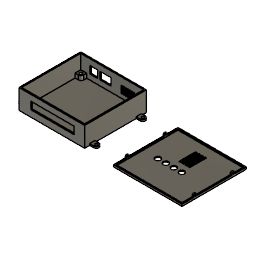
Carte ESP32 4 Relais (Autodesk Fusion 360 design; units mm, degrees)
Autodesk Fusion 360 part; units mm, degrees
note: some values were not read from the file. Chosen so that the rebuilt part matches the saved one: which bodies a step acts on; a direction. Set by a fixed rule: which sketch regions a step uses.
sketch "Esquisse1" plane through (0, 0, 0) normal (0, 0, 1) x (1, 0, 0)
  line L0 (47.5, -44.5) -> (-47.5, -44.5)
  line L1 (-47.5, -44.5) -> (-47.5, 44.5)
  line L2 (-47.5, 44.5) -> (47.5, 44.5)
  line L3 (47.5, 44.5) -> (47.5, -44.5)
  line L4 (47.5, -44.5) -> (-47.5, 44.5) construction
  line L5 (-47.5, -44.5) -> (47.5, 44.5) construction
  line L6 (49.5, -46.5) -> (-49.5, -46.5)
  line L7 (-49.5, -46.5) -> (-49.5, 46.5)
  line L8 (-49.5, 46.5) -> (49.5, 46.5)
  line L9 (49.5, 46.5) -> (49.5, -46.5)
  circle A0 centre (55.5, -35) radius 4
  line L10 (55.5, -39) -> (49.5, -39)
  line L11 (55.5, -31) -> (49.5, -31)
  circle A1 centre (55.5, 35) radius 4
  line L12 (55.5, -35) -> (55.5, 39) construction
  line L13 (60, 0) -> (0, 0) construction
  line L14 (55.5, 39) -> (49.5, 39)
  line L15 (55.5, 31) -> (49.5, 31)
  circle A2 centre (-55.5, -35) radius 4
  circle A3 centre (-55.5, 35) radius 4
  line L16 (-55.5, -35) -> (-55.5, 35) construction
  line L17 (-55.5, -39) -> (-49.5, -39)
  line L18 (-55.5, -31) -> (-49.5, -31)
  line L19 (-55.5, 31) -> (-49.5, 31)
  line L20 (-55.5, 39) -> (-49.5, 39)
  circle A4 centre (-55.5, 35) radius 2
  circle A5 centre (55.5, -35) radius 2
  circle A6 centre (-55.5, -35) radius 2
  circle A7 centre (55.5, 35) radius 2
  dimension "d1" = 95
  dimension "d2" = 89
  dimension "d3" = -2
  dimension "d56" = 8
  dimension "d59" = 8
  dimension "d60" = 70
  dimension "d61" = 8
  dimension "d62" = 8
  dimension "d63" = 6
  dimension "d64" = 6
  dimension "d65" = 4
  dimension "d66" = 4
  dimension "d67" = 4
  dimension "d68" = 4
  constraint horizontal L0
  constraint perpendicular L0 L1
  constraint parallel L0 L2
  constraint parallel L1 L3
  constraint coincident L4 L13.end
  constraint coincident L5 L13.end
  constraint coincident L13.end origin
  constraint coincident A0 L10.start
  constraint coincident L9 L10.end
  constraint perpendicular L9 L10
  constraint coincident A0 L11.start
  constraint coincident L9 L11.end
  constraint perpendicular L9 L11
  constraint coincident A0.centre L12.start
  constraint perpendicular L11 L12
  constraint coincident A1 L12.end
  constraint horizontal L13
  constraint symmetric A0 A1 L13
  constraint coincident L9 L14.end
  constraint tangent A1 L14
  constraint coincident A1 L15.start
  constraint coincident L12 L15.start
  constraint coincident L9 L15.end
  constraint perpendicular L9 L15
  constraint coincident A2.centre L16.start
  constraint coincident A3.centre L16.end
  constraint vertical L16
  constraint coincident A2 L17.start
  constraint coincident L7 L17.end
  constraint perpendicular L7 L17
  constraint coincident A2 L18.start
  constraint coincident L16 L18.start
  constraint coincident L7 L18.end
  constraint perpendicular L7 L18
  constraint coincident A3 L19.start
  constraint coincident L16 L19.start
  constraint coincident L7 L19.end
  constraint perpendicular L7 L19
  constraint coincident A3 L20.start
  constraint coincident L7 L20.end
  constraint perpendicular L7 L20
  constraint concentric A2 A6
  constraint concentric A1 A7
  measures "d1" distance of L1.end L2.end
  measures "d2" distance of L0.end L1.end
  measures "d56" diameter of A0
  measures "d59" diameter of A1
  measures "d60" distance of A0.centre A1.centre
  measures "d61" diameter of A2
  measures "d62" diameter of A3
  measures "d63" distance of L9 A0.centre
  measures "d64" distance of L7 L16
  measures "d65" diameter of A4
  measures "d66" diameter of A5
  measures "d67" diameter of A6
  measures "d68" diameter of A7
extrude "Extrusion1" add sketch "Esquisse1" along normal blind 2 contours L0 L1 L2 L3 makes body 1
extrude "Extrusion8" add sketch "Esquisse1" along normal blind 2.5 separate body contours L9 A0 L10 L11 | L7 A2 L17 L18 | A0 | A2 | L9 A1 L14 L15 | L7 A3 L19 L20 | A1 | A3 makes body 2 at (50.8333, -35, 0) makes body 3 at (50.8333, 35, 2.5) makes body 4 at (-50.8333, 35, 0) makes body 5 at (-50.8333, -35, 0)
extrude "Extrusion2" add sketch "Esquisse1" along normal blind 30 contours L6 L7 L8 L9 bodies 1 2 3 4 5
sketch "Esquisse2" plane through (0, -46.5, 0) normal (0, -1, 0) x (1, 0, 0)
  line L0 (-49.5, 0) -> (49.5, 0)
  line L1 (49.5, 0) -> (49.5, 30)
  line L2 (49.5, 30) -> (-49.5, 30)
  line L3 (-49.5, 30) -> (-49.5, 0)
  line L4 (-31.5, 0) -> (33.5, 0)
  line L5 (33.5, 0) -> (33.5, 21)
  line L6 (33.5, 21) -> (-31.5, 21)
  line L7 (-31.5, 21) -> (-31.5, 0)
  line L8 (-31.5, 10) -> (33.5, 10)
  dimension "d8" = 18
  dimension "d9" = 65
  dimension "d11" = 10
  dimension "d135" = 11
  constraint horizontal L4
  constraint vertical L5
  constraint horizontal L6
  constraint vertical L7
  constraint coincident L0 L4.start
  constraint coincident L7 L8.start
  constraint coincident L5 L8.end
  constraint perpendicular L5 L8
  measures "d8" distance of L3 L7
  measures "d9" distance of L5.end L6.end
  measures "d11" distance of L4 L8
  measures "d135" distance of L6 L8
extrude "Extrusion3" cut sketch "Esquisse2" against normal up to surface (2 mm away) contours L5 L6 L7 L8 bodies 1
sketch "Esquisse3" plane through (0, 46.5, 0) normal (0, 1, 0) x (-1, 0, 0)
  line L0 (-49.5, 0) -> (49.5, 0)
  line L1 (49.5, 0) -> (49.5, 30)
  line L2 (49.5, 30) -> (-49.5, 30)
  line L3 (-49.5, 30) -> (-49.5, 0)
  line L4 (33.5, 0) -> (2, 0)
  line L5 (2, 0) -> (2, 21)
  line L6 (2, 21) -> (33.5, 21)
  line L7 (33.5, 21) -> (33.5, 0)
  line L8 (18.5, 21) -> (22, 21)
  line L9 (22, 21) -> (22, 0)
  line L10 (22, 0) -> (18.5, 0)
  line L11 (18.5, 0) -> (18.5, 21)
  line L12 (2, 10) -> (33.5, 10)
  dimension "d14" = 16
  dimension "d18" = 3.5
  dimension "d19" = 10
  dimension "d137" = 11.5
  dimension "d138" = 16.5
  dimension "d144" = 11
  constraint horizontal L4
  constraint vertical L5
  constraint horizontal L6
  constraint vertical L7
  constraint coincident L0 L4.start
  constraint horizontal L8
  constraint vertical L9
  constraint horizontal L10
  constraint vertical L11
  constraint coincident L6 L8.start
  constraint coincident L5 L12.start
  constraint coincident L7 L12.end
  constraint perpendicular L7 L12
  measures "d14" distance of L1 L7
  measures "d18" distance of L9 L11
  measures "d19" distance of L4 L12
  measures "d137" distance of L7 L9
  measures "d138" distance of L5 L11
  measures "d144" distance of L6 L12
extrude "Extrusion4" cut sketch "Esquisse3" against normal up to surface (2 mm away) contours L5 L6 L11 L12 | L6 L7 L9 L12 bodies 1
sketch "Esquisse4" plane through (0, 0, 2) normal (0, 0, 1) x (-1, 0, 0)
  line L0 (-47.5, -44.5) -> (47.5, -44.5)
  line L1 (47.5, -44.5) -> (47.5, 44.5)
  line L2 (47.5, 44.5) -> (-47.5, 44.5)
  line L3 (31.5, 44.5) -> (31.5, 46.5)
  line L4 (31.5, 46.5) -> (-33.5, 46.5)
  line L5 (-33.5, 46.5) -> (-33.5, 44.5)
  line L6 (-47.5, 44.5) -> (-47.5, -44.5)
  circle A0 centre (-42.5, 40) radius 4
  circle A1 centre (42.5, 40) radius 4
  line L7 (0, -48) -> (0, 48) construction
  circle A2 centre (-42.5, -40) radius 4
  circle A3 centre (42.5, -40) radius 4
  line L8 (-58.0065, 0) -> (65, 0) construction
  line L9 (18.5, -44.5) -> (2, -44.5)
  line L10 (2, -44.5) -> (2, -46.5)
  line L11 (2, -46.5) -> (18.5, -46.5)
  line L12 (18.5, -46.5) -> (18.5, -44.5)
  line L13 (33.5, -44.5) -> (22, -44.5)
  line L14 (22, -44.5) -> (22, -46.5)
  line L15 (22, -46.5) -> (33.5, -46.5)
  line L16 (33.5, -46.5) -> (33.5, -44.5)
  line L17 (-33.5, 44.5) -> (31.5, 44.5)
  line L18 (42.5, -36) -> (47.5, -36)
  line L19 (38.5, -40.0091) -> (38.5102, -44.5)
  line L20 (-42.5, -36) -> (-47.5, -36)
  line L21 (-38.5, -40) -> (-38.5, -44.5)
  line L22 (-42.4542, 36.0003) -> (-47.5, 35.9425)
  line L23 (-38.5, 40.0021) -> (-38.5024, 44.5)
  line L24 (42.5, 36) -> (47.5, 36)
  line L25 (38.5, 39.9891) -> (38.4877, 44.5)
  circle A4 centre (-42.5, 40) radius 2.3
  circle A5 centre (42.5, 40) radius 2.3
  circle A6 centre (42.5, -40) radius 2.3
  circle A7 centre (-42.5, -40) radius 2.3
  dimension "d22" = 85
  dimension "d23" = 85
  dimension "d24" = 8
  dimension "d25" = 8
  dimension "d26" = 8
  dimension "d27" = 8
  dimension "d37" = 80
  dimension "d140" = 4.6
  dimension "d141" = 4.6
  dimension "d142" = 4.6
  dimension "d143" = 4.6
  constraint midpoint L7 origin
  constraint perpendicular L4 L7
  constraint symmetric A0.centre A1.centre L7
  constraint symmetric L7 A2.centre A3.centre
  constraint perpendicular L6 L8
  constraint symmetric A0.centre A2.centre L8
  constraint coincident origin L8
  constraint coincident A3 L18.start
  constraint coincident L1 L18.end
  constraint perpendicular L1 L18
  constraint coincident A3 L19.start
  constraint coincident L0 L19.end
  constraint tangent A3 L19
  constraint coincident A2 L20.start
  constraint coincident L6 L20.end
  constraint perpendicular L6 L20
  constraint coincident A2 L21.start
  constraint coincident L0 L21.end
  constraint perpendicular L0 L21
  constraint coincident A0 L22.start
  constraint coincident L6 L22.end
  constraint tangent A0 L22
  constraint coincident A0 L23.start
  constraint coincident L2 L23.end
  constraint tangent A0 L23
  constraint coincident L1 L24.end
  constraint perpendicular L1 L24
  constraint coincident A1 L25.start
  constraint coincident L2 L25.end
  constraint tangent A1 L25
  constraint coincident A1 L24.start
  constraint concentric A0 A4
  constraint concentric A1 A5
  constraint concentric A3 A6
  constraint concentric A2 A7
  measures "d22" distance of A0.centre A1.centre
  measures "d23" distance of A2.centre A3.centre
  measures "d24" diameter of A0
  measures "d25" diameter of A1
  measures "d26" diameter of A2
  measures "d27" diameter of A3
  measures "d37" distance of A0.centre A2.centre
  measures "d140" diameter of A4
  measures "d141" diameter of A7
  measures "d142" diameter of A5
  measures "d143" diameter of A6
extrude "Extrusion5" add sketch "Esquisse4" along normal blind 6.5 contours L0 L6 A2 L20 L21 | A2 | L2 L6 A0 L22 L23 | A0 | L0 L1 A3 L18 L19 | A3 | L1 L2 A1 L24 L25 | A1 bodies 1
sketch "Esquisse6" plane through (0, 46.5, 0) normal (0, 1, 0) x (-1, 0, 0)
  line L0 (2, 21) -> (18.5, 21)
  line L1 (18.5, 21) -> (18.5, 10)
  line L2 (18.5, 10) -> (2, 10)
  line L3 (2, 10) -> (2, 21)
  line L4 (33.5, 21) -> (33.5, 10)
  line L5 (33.5, 10) -> (22, 10)
  line L6 (22, 10) -> (22, 21)
  line L7 (22, 21) -> (33.5, 21)
  line L8 (-49.5, 0) -> (49.5, 0)
  line L9 (49.5, 0) -> (49.5, 30)
  line L10 (49.5, 30) -> (-49.5, 30)
  line L11 (-49.5, 30) -> (-49.5, 0)
  line L12 (-33.5, 19) -> (-13.58, 19)
  line L13 (-13.58, 19) -> (-13.58, 8)
  line L14 (-13.58, 8) -> (-33.5, 8)
  line L15 (-33.5, 8) -> (-33.5, 19)
  line L16 (-32, 19) -> (-30.43, 19)
  line L17 (-30.43, 19) -> (-30.43, 8)
  line L18 (-30.43, 8) -> (-32, 8)
  line L19 (-32, 8) -> (-32, 19)
  line L20 (-28.93, 19) -> (-27.36, 19)
  line L21 (-27.36, 19) -> (-27.36, 8)
  line L22 (-27.36, 8) -> (-28.93, 8)
  line L23 (-28.93, 8) -> (-28.93, 19)
  line L24 (-25.86, 19) -> (-24.29, 19)
  line L25 (-24.29, 19) -> (-24.29, 8)
  line L26 (-24.29, 8) -> (-25.86, 8)
  line L27 (-25.86, 8) -> (-25.86, 19)
  line L28 (-22.79, 19) -> (-21.22, 19)
  line L29 (-21.22, 19) -> (-21.22, 8)
  line L30 (-21.22, 8) -> (-22.79, 8)
  line L31 (-22.79, 8) -> (-22.79, 19)
  line L32 (-19.72, 19) -> (-18.15, 19)
  line L33 (-18.15, 19) -> (-18.15, 8)
  line L34 (-18.15, 8) -> (-19.72, 8)
  line L35 (-19.72, 8) -> (-19.72, 19)
  line L36 (-16.65, 19) -> (-15.08, 19)
  line L37 (-15.08, 19) -> (-15.08, 8)
  line L38 (-15.08, 8) -> (-16.65, 8)
  line L39 (-16.65, 8) -> (-16.65, 19)
  dimension "d38" = 16
  dimension "d40" = 11
  dimension "d41" = 8
  dimension "d42" = 1.57
  dimension "d43" = 1.57
  dimension "d44" = 1.57
  dimension "d45" = 1.57
  dimension "d46" = 1.57
  dimension "d47" = 1.57
  dimension "d48" = 1.5
  dimension "d49" = 1.5
  dimension "d50" = 1.5
  dimension "d51" = 1.5
  dimension "d52" = 1.5
  dimension "d53" = 1.5
  dimension "d136" = 1.5
  constraint horizontal L12
  constraint vertical L13
  constraint horizontal L14
  constraint vertical L15
  constraint horizontal L16
  constraint vertical L17
  constraint horizontal L18
  constraint vertical L19
  constraint coincident L14 L17.end
  constraint coincident L12 L16.start
  constraint horizontal L20
  constraint vertical L21
  constraint horizontal L22
  constraint vertical L23
  constraint coincident L14 L21.end
  constraint coincident L12 L20.start
  constraint horizontal L24
  constraint vertical L25
  constraint horizontal L26
  constraint vertical L27
  constraint coincident L14 L25.end
  constraint coincident L12 L24.start
  constraint horizontal L28
  constraint vertical L29
  constraint horizontal L30
  constraint vertical L31
  constraint coincident L14 L29.end
  constraint coincident L12 L28.start
  constraint horizontal L32
  constraint vertical L33
  constraint horizontal L34
  constraint vertical L35
  constraint coincident L14 L33.end
  constraint horizontal L36
  constraint vertical L37
  constraint horizontal L38
  constraint vertical L39
  constraint coincident L14 L37.end
  constraint coincident L12.end L32
  constraint coincident L12.end L36
  measures "d38" distance of L11 L15
  measures "d40" distance of L12.start L14.end
  measures "d41" distance of L8 L14
  measures "d42" distance of L16.start L16.end
  measures "d43" distance of L21 L23
  measures "d44" distance of L25 L27
  measures "d45" distance of L29 L31
  measures "d46" distance of L33 L35
  measures "d47" distance of L37 L39
  measures "d48" distance of L15 L19
  measures "d49" distance of L17 L23
  measures "d50" distance of L21 L27
  measures "d51" distance of L25 L31
  measures "d52" distance of L29 L35
  measures "d53" distance of L33 L39
  measures "d136" distance of L13 L37
extrude "Extrusion7" cut sketch "Esquisse6" against normal up to surface (2 mm away) contours L12 L14 L15 L19 | L12 L14 L17 L23 | L12 L14 L21 L27 | L12 L14 L25 L31 | L12 L14 L29 L35 | L12 L14 L33 L39 | L12 L13 L14 L37 bodies 1
sketch "Esquisse8" plane through (0, 0, 2) normal (0, 0, 1) x (-1, 0, 0)
  line L0 (-38.5, -44.5) -> (38.5102, -44.5)
  line L1 (47.5, -36) -> (47.5, 36)
  line L2 (38.4877, 44.5) -> (-38.5024, 44.5)
  line L3 (-47.5, 35.9425) -> (-47.5, -36)
  line L4 (-99.3796, -44.1687) -> (-198.5796, -44.1687)
  line L5 (-198.5796, -44.1687) -> (-198.5796, 49.0313)
  line L6 (-198.5796, 49.0313) -> (-99.3796, 49.0313)
  line L7 (-99.3796, 49.0313) -> (-99.3796, -44.1687)
  line L8 (-200.5796, 51.0313) -> (-97.3796, 51.0313)
  line L9 (-97.3796, 51.0313) -> (-97.3796, -46.1687)
  line L10 (-97.3796, -46.1687) -> (-200.5796, -46.1687)
  line L11 (-200.5796, -46.1687) -> (-200.5796, 51.0313)
  line L12 (42.5012, -36) -> (47.5, -36)
  line L13 (38.5102, -44.5) -> (38.5, -40.0091)
  arc A0 (42.5012, -36) -> (38.5, -40.0091) centre (42.5, -40) ccw
  line L14 (47.5, 36) -> (42.5, 36)
  arc A1 (38.5, 39.9891) -> (42.5, 36) centre (42.5, 40) ccw
  line L15 (38.5, 39.9891) -> (38.4877, 44.5)
  line L16 (-38.5024, 44.5) -> (-38.5, 40.0021)
  arc A2 (-42.4542, 36.0003) -> (-38.5, 40.0021) centre (-42.5, 40) ccw
  line L17 (-42.4542, 36.0003) -> (-47.5, 35.9425)
  line L18 (-47.5, -36) -> (-42.5, -36)
  arc A3 (-38.5, -40.0012) -> (-42.5, -36) centre (-42.5, -40) ccw
  line L19 (-38.5, -40.0012) -> (-38.5, -44.5)
  dimension "d69" = 99.2
  dimension "d70" = 93.2
  dimension "d71" = -2
  constraint horizontal L4
  constraint vertical L5
  constraint horizontal L6
  constraint vertical L7
  measures "d69" distance of L4.start L4.end
  measures "d70" distance of L4.start L6.end
extrude "Extrusion9" add sketch "Esquisse8" along normal blind 1.5 separate body contours L4 L5 L6 L7 makes body 6
extrude "Extrusion10" add sketch "Esquisse8" along normal blind 3 contours L8 L9 L10 L11 bodies 6
sketch "Esquisse9" plane through (200.5796, 0, 0) normal (1, 0, 0) x (0, 1, 0)
  line L0 (-51.0313, 2) -> (46.1687, 2)
  line L1 (46.1687, 2) -> (46.1687, 5)
  line L2 (46.1687, 5) -> (-51.0313, 5)
  line L3 (-51.0313, 5) -> (-51.0313, 2)
  circle A0 centre (26.1687, 6.5) radius 2.5
  line L4 (46.1687, 2) -> (-51.0313, 2)
  line L5 (23.6687, 6.5) -> (23.6687, 5)
  line L6 (28.6687, 6.5) -> (28.6687, 5)
  circle A1 centre (-31.0313, 6.5) radius 2.5
  line L7 (-28.5313, 6.5) -> (-28.5313, 5)
  line L8 (-33.5313, 6.5) -> (-33.5313, 5)
  line L9 (-51.0313, 2) -> (46.1687, 2)
  line L10 (46.1687, 2) -> (46.1687, 5)
  line L11 (46.1687, 5) -> (-51.0313, 5)
  line L12 (-51.0313, 5) -> (-51.0313, 2)
  point P0 (-40, 2)
  dimension "d76" = 5
  dimension "d77" = 4.5
  dimension "d80" = 5
  dimension "d81" = 4.5
  dimension "d82" = 20
  dimension "d83" = 20
  constraint coincident A0 L5.start
  constraint coincident L2 L5.end
  constraint tangent A0 L5
  constraint perpendicular L2 L5
  constraint coincident A0 L6.start
  constraint coincident L2 L6.end
  constraint tangent A0 L6
  constraint coincident A1 L7.start
  constraint coincident L2 L7.end
  constraint tangent A1 L7
  constraint coincident A1 L8.start
  constraint coincident L2 L8.end
  constraint tangent A1 L8
  constraint vertical L7
  constraint vertical L8
  constraint vertical L6
  measures "d76" diameter of A0
  measures "d77" distance of A0.centre L4
  measures "d80" diameter of A1
  measures "d81" vertical distance of A1.centre P0
  measures "d82" distance of L1 A0.centre
  measures "d83" distance of L3 A1.centre
extrude "Extrusion11" add sketch "Esquisse9" against normal up to surface (2 mm away) contours L2 A1 L8 L11 | L2 A0 L6 L11 | L2 A1 L11 | L2 A1 L11 | L2 A0 L11 | L2 A0 L11 | L2 A1 L7 L11 | L2 A0 L5 L11 bodies 6
hole "Perçage3" at (200.5796, -31.0313, 6.5) at (200.5796, 26.1687, 6.5) direction (-1, 0, 0) diameter 2 depth 11 tip angle 118 countersink diameter 3 countersink angle 90 bodies 6
sketch "Esquisse10" plane through (97.3796, 0, 0) normal (-1, 0, 0) x (0, -1, 0)
  line L0 (-46.1687, 2) -> (51.0313, 2)
  line L1 (51.0313, 2) -> (51.0313, 5)
  line L2 (51.0313, 5) -> (-46.1687, 5)
  line L3 (-46.1687, 5) -> (-46.1687, 2)
  circle A0 centre (-26.1687, 6.5) radius 2.5
  line L4 (51.0313, 2) -> (-46.1687, 2)
  line L5 (-28.6687, 6.5016) -> (-28.6697, 5)
  line L6 (-23.6687, 6.5016) -> (-23.6678, 5)
  circle A1 centre (31.0313, 6.5) radius 2.5
  line L7 (28.5313, 6.5077) -> (28.5267, 5)
  line L8 (33.5313, 6.5077) -> (33.5359, 5)
  dimension "d99" = 5
  dimension "d100" = 4.5
  dimension "d101" = 20
  dimension "d102" = 5
  dimension "d103" = 4.5
  dimension "d104" = 20
  constraint coincident A0 L5.start
  constraint coincident L2 L5.end
  constraint tangent A0 L5
  constraint coincident A0 L6.start
  constraint coincident L2 L6.end
  constraint tangent A0 L6
  constraint coincident A1 L7.start
  constraint coincident L2 L7.end
  constraint tangent A1 L7
  constraint coincident A1 L8.start
  constraint coincident L2 L8.end
  constraint tangent A1 L8
  measures "d99" diameter of A0
  measures "d100" distance of A0.centre L4
  measures "d101" distance of L3 A0.centre
  measures "d102" diameter of A1
  measures "d103" distance of L4 A1.centre
  measures "d104" distance of L1 A1.centre
extrude "Extrusion12" add sketch "Esquisse10" against normal up to surface (2 mm away) contours L2 A0 L5 | L2 A1 L8 | L2 A0 | L2 A1 L8 | L2 A0 L6 | L2 A1 L7 picked at (-26.9468, 6.6584) bodies 6
hole "Perçage4" at (97.3796, 26.1687, 6.5) at (97.3796, -31.0313, 6.5) direction (1, 0, 0) diameter 2 depth 11 tip angle 118 countersink diameter 3 countersink angle 90 bodies 6
sketch "Esquisse11" plane through (0, 0, 3.5) normal (0, 0, 1) x (-1, 0, 0)
  line L0 (-99.3796, 49.0313) -> (-198.5796, 49.0313)
  line L1 (-198.5796, 49.0313) -> (-198.5796, -44.1687)
  line L2 (-198.5796, -44.1687) -> (-99.3796, -44.1687)
  line L3 (-99.3796, -44.1687) -> (-99.3796, 49.0313)
  line L4 (-157.0796, -29.1687) -> (-154.5796, -29.1687)
  line L5 (-154.5796, -29.1687) -> (-154.5796, -4.1687)
  line L6 (-154.5796, -4.1687) -> (-157.0796, -4.1687)
  line L7 (-157.0796, -4.1687) -> (-157.0796, -29.1687)
  line L8 (-152.5796, -29.1687) -> (-150.0796, -29.1687)
  line L9 (-150.0796, -29.1687) -> (-150.0796, -4.1687)
  line L10 (-150.0796, -4.1687) -> (-152.5796, -4.1687)
  line L11 (-152.5796, -4.1687) -> (-152.5796, -29.1687)
  line L12 (-148.0796, -29.1687) -> (-145.5796, -29.1687)
  line L13 (-145.5796, -29.1687) -> (-145.5796, -4.1687)
  line L14 (-145.5796, -4.1687) -> (-148.0796, -4.1687)
  line L15 (-148.0796, -4.1687) -> (-148.0796, -29.1687)
  line L16 (-143.5796, -29.1687) -> (-141.0796, -29.1687)
  line L17 (-141.0796, -29.1687) -> (-141.0796, -4.1687)
  line L18 (-141.0796, -4.1687) -> (-143.5796, -4.1687)
  line L19 (-143.5796, -4.1687) -> (-143.5796, -29.1687)
  line L20 (-148.9796, -44.1687) -> (-148.9796, 49.0313) construction
  circle A0 centre (-121.3796, 8.0313) radius 4
  circle A1 centre (-133.3796, 8.0313) radius 4
  circle A2 centre (-145.3796, 8.0313) radius 4
  circle A3 centre (-157.3796, 8.0313) radius 4
  line L21 (-160, 8.0313) -> (-121.3796, 8.0313) construction
  dimension "d112" = 2.5
  dimension "d113" = 2.5
  dimension "d114" = 2.5
  dimension "d115" = 2.5
  dimension "d116" = 2
  dimension "d117" = 2
  dimension "d118" = 2
  dimension "d119" = 15
  dimension "d120" = 25
  dimension "d121" = 25
  dimension "d122" = 25
  dimension "d123" = 25
  dimension "d124" = 41.5
  dimension "d126" = 8
  dimension "d127" = 22
  dimension "d128" = 8
  dimension "d129" = 8
  dimension "d130" = 8
  dimension "d131" = 12
  dimension "d132" = 12
  dimension "d133" = 12
  dimension "d134" = 41
  constraint horizontal L4
  constraint vertical L5
  constraint horizontal L6
  constraint vertical L7
  constraint horizontal L8
  constraint vertical L9
  constraint horizontal L10
  constraint vertical L11
  constraint horizontal L12
  constraint vertical L13
  constraint horizontal L14
  constraint vertical L15
  constraint horizontal L16
  constraint vertical L17
  constraint horizontal L18
  constraint vertical L19
  constraint coincident L2 L20.start
  constraint coincident L0 L20.end
  constraint perpendicular L0 L20
  constraint symmetric L1 L3 L20
  constraint horizontal L21
  constraint coincident A0.centre L21.end
  constraint coincident A1.centre L21
  constraint coincident A2.centre L21
  constraint coincident A3.centre L21
  measures "d112" distance of L4.start L4.end
  measures "d113" distance of L8.start L8.end
  measures "d114" distance of L12.start L12.end
  measures "d115" distance of L16.start L16.end
  measures "d116" distance of L5 L11
  measures "d117" distance of L9 L15
  measures "d118" distance of L13 L19
  measures "d119" distance of L2 L4
  measures "d120" distance of L4.start L6.end
  measures "d121" distance of L8.start L10.end
  measures "d122" distance of L12.start L14.end
  measures "d123" distance of L16.start L18.end
  measures "d124" distance of L1 L7
  measures "d126" diameter of A0
  measures "d127" distance of L3 A0.centre
  measures "d128" diameter of A1
  measures "d129" diameter of A2
  measures "d130" diameter of A3
  measures "d131" distance of A0.centre A1.centre
  measures "d132" distance of A1.centre A2.centre
  measures "d133" distance of A2.centre A3.centre
  measures "d134" distance of L0 A0.centre
extrude "Extrusion13" cut sketch "Esquisse11" against normal through all contours L4 L5 L6 L7 | L8 L9 L10 L11 | L12 L13 L14 L15 | L16 L17 L18 L19 | A0 | A1 | A2 | A3 bodies 6
equation "d25 = d24"
equation "d26 = d24"
equation "d27 = d24"
equation "d43 = d42"
equation "d44 = d42"
equation "d45 = d42"
equation "d46 = d42"
equation "d47 = d42"
equation "d49 = d48"
equation "d50 = d48"
equation "d51 = d48"
equation "d52 = d48"
equation "d53 = d48"
equation "d59 = d56"
equation "d61 = d56"
equation "d62 = d56"
equation "d64 = d63"
equation "d65 = d66"
equation "d67 = d66"
equation "d68 = d66"
equation "d69 = d1 - ( 2 * d3 ) + 0.2 mm"
equation "d70 = d2 - ( 2 * d3 ) + 0.2 mm"
equation "d80 = d76"
equation "d81 = d77"
equation "d83 = d82"
equation "d99 = d76"
equation "d100 = d77"
equation "d101 = d82"
equation "d102 = d76"
equation "d103 = d77"
equation "d104 = d82"
equation "d113 = d112"
equation "d114 = d112"
equation "d115 = d112"
equation "d117 = d116"
equation "d118 = d116"
equation "d121 = d120"
equation "d122 = d120"
equation "d123 = d120"
equation "d128 = d126"
equation "d129 = d126"
equation "d130 = d126"
equation "d132 = d131"
equation "d133 = d131"
equation "d136 = d48"
equation "d141 = d140"
equation "d142 = d140"
equation "d143 = d140"
named bodies: "Boitier", "Couvercle"
